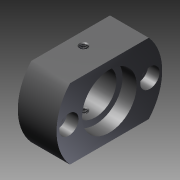
# Autodesk Inventor part: BGCSB12_h
Saved by Autodesk Inventor 2011 SP1 (Build 150282100, 282)
## iProperties
Created: 2016-11-09
Part Number: BGCSB12_h
Catalog Web Link: www.cadenas.de
Description: BGCSB, BGCS, SBGCS_housing-Bearing with Housings - Thrust Bearings - Standard
Vendor: MISUMI
Document SubType Name: Modeling
Designer: psAdmin
Manufacturer: MISUMI
Mass: 33.6519 g
Surface Area: 103.159 cm^2
Volume: 33.6519 cm^3
Density: 1 g/cm^3
Category: PARTsolutions
Company: MISUMI
Title: BGCSB12
Author: Cadenas PARTsolutions
Comments: Bearing with Housings - Thrust Bearings - Standard
PSOL_IDENT_0: {$CADENAS_DATA\23d-libs\misumi\metric\12_bearing_holders\bgcsb\housing_bgcsb.prj},184 {VTYP=3D},{NB=
PSOL_IDENT_1: BGCSB12_h},{LINA=BGCSB12},{NN=BGCSB, BGCS, SBGCS_housing},{DATE=17.06.2016 05:47:01},{GEOMDATE=02.03
PSOL_IDENT_2: .2016 00:34:00},{VERSION=},{LINEID=30},{LINESUBID=-1},{WBVAR=MAT,ST}  {NB=BGCSB12_h},{LINA=BGCSB12},
PSOL_IDENT_3: {KT=DUMMY},{PN=BGCSB12},{TYPE=BGCSB},{MAT=BG},{MAT1= 'BG','S45C Equivalent','SBG','SUS304' },{ST=B},
PSOL_IDENT_4: {ST1=    'B','Black Oxide','ENP','Electroless Nickel Plating'               },{DD=12},{D=24},{B=23},
PSOL_IDENT_5: {H=60},{W=40},{T=22},{DDZZ=15},{D1=29},{D2=31},{D3=30},{T1=14},{B1=15.5},{A=46},{F=0},{M=M8 (6.8)},{
PSOL_IDENT_6: DD1=11},{H1=6.5},{BN=NKXZ12},{DD2=6.800},{MMAX=8.000},{M1=5},{M1L=8}
NN: BGCSB, BGCS, SBGCS_housing
NT: Bearing with Housings - Thrust Bearings - Standard
NB: BGCSB12_h
NBSYN: $PN._h
LINA: BGCSB12
PN: BGCSB12
MAT: S45C Equivalent
ST: Black Oxide
DD: 12
D: 24
B: 23
H: 60
W: 40
T: 22
DDZZ: 15
D1: 29
D2: 31
D3: 30
T1: 14
B1: 15.5
A: 46
F: 0
M: M8 (6.8)
DD1: 11
H1: 6.5
BN: NKXZ12
SUPPLIER: MISUMI
ARTICLENO: BGCSB12_h
BOMINFO: BGCSB12
CREATOR: CADENAS GmbH
Autodesk Inventor part; units mm, degrees
ref_plane "YZ Plane" through (0, 0, 0) normal (1, 0, 0) x (0, 1, 0)
ref_plane "XZ Plane" through (0, 0, 0) normal (0, 1, 0) x (-1, 0, 0)
ref_plane "XY Plane" through (0, 0, 0) normal (0, 0, 1) x (1, 0, 0)
sketch "Sketch_1" plane through (0, 0, 0) normal (0, 0, 1) x (1, 0, 0)
  line L0 (22, 0) -> (0, 0)
  line L1 (0, 30) -> (0, 12)
  line L2 (0, 12) -> (14, 12)
  line L3 (14, 12) -> (14, 15.5)
  line L4 (14, 15.5) -> (22, 15.5)
  line L5 (22, 15.5) -> (22, 30)
  line L6 (22, 30) -> (0, 30)
  constraints: 14 end point
revolve "Revolution1" add sketch "Sketch_1" angle 360 about axis through (22, 0, 0) along (1, 0, 0)
sketch "Sketch_2" plane through (0, 0, 0) normal (1, 0, 0) x (0, 1, 0)
  line L0 (-120, 80) -> (-120, -80)
  line L1 (-120, -80) -> (120, -80)
  line L2 (120, -80) -> (120, 80)
  line L3 (120, 80) -> (-120, 80)
  line L4 (-30, 20) -> (-30, -20)
  line L5 (-30, -20) -> (30, -20)
  line L6 (30, -20) -> (30, 20)
  line L7 (30, 20) -> (-30, 20)
  constraints: 16 end point
extrude "Extrusion1" cut sketch "Sketch_2" along normal blind 24
sketch "Sketch_3" plane through (0, 0, 0) normal (0, 0, 1) x (1, 0, 0)
  line L0 (22, 23) -> (0, 23)
  line L1 (0, 23) -> (0, 27)
  line L2 (0, 27) -> (0.6765, 26.3235)
  line L3 (0.6765, 26.3235) -> (14.8235, 26.3235)
  line L4 (14.8235, 26.3235) -> (15.5, 27)
  line L5 (15.5, 27) -> (15.5, 28.5)
  line L6 (15.5, 28.5) -> (22, 28.5)
  line L7 (22, 28.5) -> (22, 23)
  line L8 (22, 23) -> (0, 23)
  constraints: 18 end point
revolve "Revolution2" cut sketch "Sketch_3" angle 360 about axis through (22, 23, 0) along (1, 0, 0)
thread "Thread1" size "M8x1.25" class "6H" standard "ISO Metric profile" full length
pattern_linear "Rectangular Pattern1" count 2 spacing 46 along (0, -1, 0) of "Revolution2"
sketch "Sketch_4" plane through (7.5, 0, 0) normal (1, 0, 0) x (0, 0, -1)
  line L0 (-11.65, 0) -> (-20, 0)
  line L1 (-20, 0) -> (-20, 2.5)
  line L2 (-20, 2.5) -> (-19.567, 2.067)
  line L3 (-19.567, 2.067) -> (-12.083, 2.067)
  line L4 (-12.083, 2.067) -> (-11.65, 2.5)
  line L5 (-11.65, 2.5) -> (-11.65, 0)
  line L6 (-11.65, 0) -> (-20, 0)
  constraints: 14 end point
revolve "Revolution3" cut sketch "Sketch_4" angle 360 about axis through (7.5, 0, 11.65) along (0, 0, -1)
thread "Thread2" size "M5x0.8" class "6H" standard "ISO Metric profile" full length
sketch "Sketch_6" plane through (7.5, 0, 0) normal (1, 0, 0) x (0, 0, -1)
  line L0 (20, 0) -> (11.65, 0)
  line L1 (11.65, 0) -> (11.65, 2.5)
  line L2 (11.65, 2.5) -> (12.083, 2.067)
  line L3 (12.083, 2.067) -> (19.567, 2.067)
  line L4 (19.567, 2.067) -> (20, 2.5)
  line L5 (20, 2.5) -> (20, 0)
  line L6 (20, 0) -> (11.65, 0)
  constraints: 14 end point
revolve "Revolution4" cut sketch "Sketch_6" angle 360 about axis through (7.5, 0, -20) along (0, 0, -1)
thread "Thread3" size "M5x0.8" class "6H" standard "ISO Metric profile" full length
ref_plane "to_bearings_XY" through (14, 0, 0) normal (1, 0, 0) x (0, 0, -1)
ref_plane "to_bearings_YZ" through (14, 0, 0) normal (0, 0, -1) x (0, 1, 0)
ref_plane "to_bearings_ZX" through (14, 0, 0) normal (0, 1, 0) x (1, 0, 0)
ref_plane "to_screw1_XY" through (7.5, 0, 12) normal (0, 0, 1) x (1, 0, 0)
ref_plane "to_screw1_YZ" through (7.5, 0, 12) normal (1, 0, 0) x (0, 1, 0)
ref_plane "to_screw1_ZX" through (7.5, 0, 12) normal (0, 1, 0) x (0, 0, 1)
ref_plane "to_screw2_XY" through (7.5, 0, -12) normal (0, 0, -1) x (1, 0, 0)
ref_plane "to_screw2_YZ" through (7.5, 0, -12) normal (1, 0, 0) x (0, -1, 0)
ref_plane "to_screw2_ZX" through (7.5, 0, -12) normal (0, -1, 0) x (0, 0, -1)
body "Solid1"
